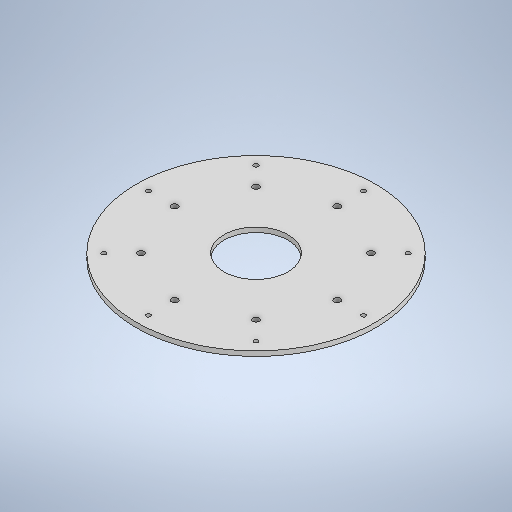
# Autodesk Inventor part: DMF pancake
Saved by Autodesk Inventor 2025 (Build 290162010, 162A)
## iProperties
Created: 2025-08-21
Part Number: DMF pancake
Material: Generic
Document SubType Name: Sheet Metal
Designer: pokla
Density: 1 g/cm^3
Appearance: Default
Flat Pattern Width: 50 cm
Flat Pattern Length: 50 cm
Flat Pattern Area: 2500 cm^2
Sheet Metal Rule: Default_mm
Sheet Metal Width: 500,000 mm
Sheet Metal Length: 500,000 mm
Sheet Metal Area: 250000,000 mm^2
Author: pokla
Autodesk Inventor part; units mm, degrees
ref_plane "YZ Plane" through (0, 0, 0) normal (1, 0, 0) x (0, 1, 0)
ref_plane "XZ Plane" through (0, 0, 0) normal (0, 1, 0) x (-1, 0, 0)
ref_plane "XY Plane" through (0, 0, 0) normal (0, 0, 1) x (1, 0, 0)
sketch "Sketch1" plane through (0, 0, 0) normal (0, 0, 1) x (1, 0, 0)
  circle A0 centre (0, 0) radius 67
  circle A1 centre (0, 0) radius 250
  dimension "d0" = 134
  dimension "d1" = 500
  constraints: 2 centre point, 2 coincident
  measures "d0" diameter of A0
  measures "d1" diameter of A1
extrude "Extrusion1" add sketch "Sketch1" along normal blind 10
sketch "Sketch2" plane through (0, 0, 10) normal (0, 0, 1) x (1, 0, 0)
  circle A0 centre (0, 0) radius 225 construction
  circle A1 centre (0, 0) radius 250 projected
  point P0 (0, 225)
  dimension "d4" = 450
  constraints: 2 vertical alignment, 1 coincident, 2 other
hole "Hole1" at (0, 225, 10) direction (0, 0, -1) diameter 9 end through all
pattern_circular "Circular Pattern1" count 8 over 360 about axis through (0, 0, 0) along (0, 0, 1) of "Hole1"
sketch "Sketch3" plane through (0, 0, 10) normal (0, 0, 1) x (1, 0, 0)
  circle A0 centre (0, 0) radius 170 construction
  point P0 (0, 170)
  dimension "d16" = 340
  constraints: 2 vertical alignment, 1 coincident, 2 other
hole "Hole2" at (0, 170, 10) direction (0, 0, -1) diameter 13 end through all
pattern_circular "Circular Pattern2" count 8 over 360 about axis through (0, 0, -10) along (0, 0, 1) of "Hole2"
equation "\"d22\" = Thickness"
equation "\"BendRadius\" = Thickness"
equation "\"BendReliefWidth\" = Thickness"
equation "\"BendReliefDepth\" = 0.5 * Thickness"
equation "\"CornerReliefSize\" = 4 * Thickness"
equation "\"MinimumRemnant\" = 2 * Thickness"
equation "\"TransitionRadius\" = BendRadius"
equation "\"JacobiRadiusSize\" = BendRadius"
equation "\"GapSize\" = Thickness"
equation "\"Thickness\" = 0.5"
body "Solid1"
